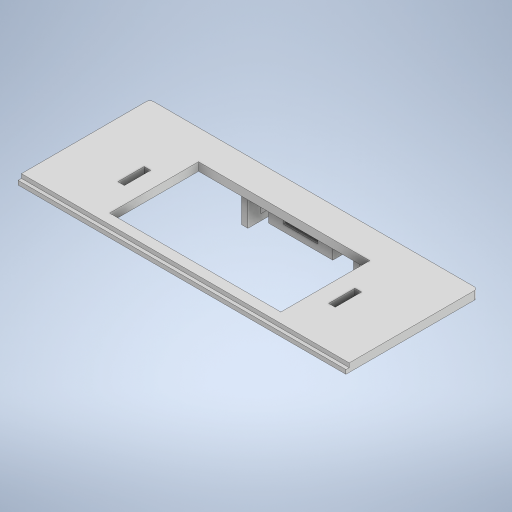
# Autodesk Inventor part: Kryt těla
Saved by Autodesk Inventor 2023 (Build 270158000, 158)
## iProperties
Created: 2023-03-18
Part Number: Kryt těla
Material: Všeobecné
Document SubType Name: Modeling
Designer: jaryj
Density: 1 g/cm^3
Appearance: Výchozí
Author: jaryj
Autodesk Inventor part; units mm, degrees
ref_plane "YZ Plane" through (0, 0, 0) normal (1, 0, 0) x (0, 1, 0)
ref_plane "XZ Plane" through (0, 0, 0) normal (0, 1, 0) x (-1, 0, 0)
ref_plane "XY Plane" through (0, 0, 0) normal (0, 0, 1) x (1, 0, 0)
sketch "Náčrt1" plane through (0, 0, 0) normal (0, 1, 0) x (-1, 0, 0)
  line L0 (0, 0) -> (49.75, 0)
  line L1 (49.75, 0) -> (49.75, -40)
  line L2 (49.75, -40) -> (0, -40)
  line L3 (0, -1) -> (49.75, -1)
  line L4 (18, -36) -> (16, -36)
  line L5 (18, -36) -> (18, -39.9)
  line L6 (18, -39.9) -> (16, -39.9)
  line L7 (16, -39.9) -> (16, -36)
  line L8 (5.25, -40) -> (5.25, -36)
  line L9 (5.25, -36) -> (9.75, -36)
  line L10 (9.75, -36) -> (9.75, -40)
  line L11 (0, -4) -> (26, -4)
  line L12 (26, -4) -> (26, -31)
  line L13 (26, -31) -> (0, -31)
  line L14 (0, -40) -> (0, -31)
  line L15 (0, -4) -> (0, 0)
  line L16 (33, -13.5) -> (31, -13.5)
  line L17 (31, -13.5) -> (31, -21.5)
  line L18 (31, -21.5) -> (33, -21.5)
  line L19 (33, -21.5) -> (33, -13.5)
  point P0 (49.75, -20)
  point P1 (33, -17.5)
  point P2 (26, -17.5)
  dimension "d0" = 40
  dimension "d1" = 49.75
  dimension "d2" = 1
  dimension "d5" = 4
  dimension "d16" = 0.1
  dimension "d17" = 31.75
  dimension "d18" = 2
  dimension "d28" = 4.5
  dimension "d29" = 4
  dimension "d57" = 27
  dimension "d58" = 26
  dimension "d59" = 5.25
  dimension "d60" = 8
  dimension "d61" = 2
  dimension "d62" = 5
  dimension "d63" = 4
  constraints: 40 end point, 11 perpendicular, 6 parallel, 4 point on line, 3 horizontal, 3 midpoint, 1 horizontal alignment, 1 vertical
  measures "d0" distance of L2.end L0.start
  measures "d1" distance of L1.end L2.end
  measures "d2" distance between parallel lines of L0 L3
  measures "d5" distance between parallel lines of L2 L4
  measures "d16" distance between parallel lines of L2 L6
  measures "d17" distance from line of L1 L4.start
  measures "d18" distance of L4.start L4.end
  measures "d28" distance of L8.end L9.end
  measures "d29" distance of L9.end L10.end
  measures "d57" distance of L11.end L12.end
  measures "d58" distance of L11.start L11.end
  measures "d59" distance between parallel lines of L14 L8
  measures "d60" distance of L18.end L16.start
  measures "d61" distance of L16.start L16.end
  measures "d62" distance between parallel lines of L12 L17
  measures "d63" distance of L11.start L0.start
extrude "Vysunutí1" add sketch "Náčrt1" along normal blind 2.5 contours L3 L1 L2 L10 L9 L8 L14 L13 L12 L11 L15 | L2 L8 L9 L10 | L5 L6 L7 L4
extrude "Vysunutí2" add sketch "Náčrt1" along normal blind 1.25 contours L0 L1 L3 L15
extrude "Vysunutí3" add sketch "Náčrt1" against normal blind 12.5 contours L5 L6 L7 L4
sketch "Náčrt3" plane through (-16, 0, -39.9) normal (0, 0, -1) x (-1, 0, 0)
  line L0 (0, 0) -> (0, -12.5) projected
  line L1 (0, -12.5) -> (2, -12.5) projected
  line L2 (2, 0) -> (2, -12.5) projected
  line L3 (0, 0) -> (0, -12.5) projected
  line L4 (0, -10.6) -> (2, -10.6)
  line L5 (2, 0) -> (2, -12.5) projected
  point P0 (-16, 0)
  point P1 (2, -10.6)
  point P2 (0, -10.6)
  dimension "d19" = 1.9
  constraints: 2 end point, 2 point on line, 1 perpendicular
  measures "d19" distance between parallel lines of L4 L1
extrude "Vysunutí5" add sketch "Náčrt3" along normal blind 5
fillet "Zaoblení1" radius 1 1 edges at (-49.75, 1.25, -40)
extrude "Vysunutí6" add sketch "Náčrt1" against normal blind 8 contours L2 L8 L9 L10
sketch "Náčrt7" plane through (-5.25, -8, -36) normal (1, 0, 0) x (0, 0, -1)
  line L0 (0, 8) -> (0, 0) projected
  line L1 (0, 0) -> (4, 0) projected
  line L2 (4, 8) -> (4, 0) projected
  line L3 (0, 8) -> (0, 0) projected
  line L4 (0, 2) -> (4, 2)
  line L5 (4, 8) -> (4, 0) projected
  point P0 (-36, 8)
  dimension "d36" = 2
  constraints: 2 end point, 2 point on line, 1 perpendicular
  measures "d36" distance between parallel lines of L1 L4
extrude "Vysunutí8" add sketch "Náčrt7" along normal up to surface (5.25 mm away)
sketch "Náčrt8" plane through (0, 0, -40) normal (0, 0, -1) x (-1, 0, 0)
  line L0 (9.75, 0) -> (9.75, -8) projected
  line L1 (5.25, -6) -> (0, -6) projected
  point P0 (0, 0)
  point P1 (7.5, -3)
  dimension "d46" = 2.25
  dimension "d47" = 3
  measures "d46" distance from line of L0 point (7.5, -3)
  measures "d47" distance from line of L1 point (7.5, -3)
hole "Díra1" at (-7.5, -3, -40) direction (0, 0, 1) diameter 2 end through all
mirror "Zrcadlit2" about plane through (0, 0, -40) normal (1, 0, 0)
